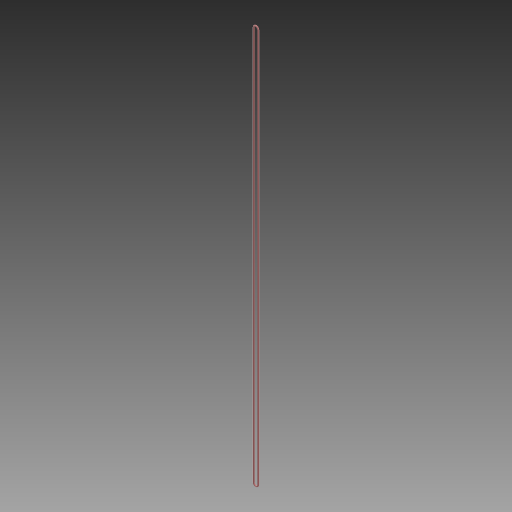
# Autodesk Inventor part: REVLIFT-Test String
Saved by Autodesk Inventor 2023 (Build 270158000, 158)
## iProperties
Created: 2023-01-02
Part Number: REVLIFT-Test String
Material: Nylon 6
Document SubType Name: Modeling
Designer: Max Boord
Mass: 32.7487 g
Surface Area: 292.399 cm^2
Volume: 29.2399 cm^3
Density: 1.12 g/cm^3
Appearance: Smooth - Burnt Red
Author: Max Boord
Autodesk Inventor part; units mm, degrees
ref_plane "YZ Plane" through (0, 0, 0) normal (1, 0, 0) x (0, 1, 0)
ref_plane "XZ Plane" through (0, 0, 0) normal (0, 1, 0) x (-1, 0, 0)
ref_plane "XY Plane" through (0, 0, 0) normal (0, 0, 1) x (1, 0, 0)
sketch "Sketch1" plane through (0, 0, 0) normal (0, 0, 1) x (1, 0, 0)
  line L0 (0, 571.5) -> (0, -571.5) construction
  line L1 (-6.5, 571.5) -> (-6.5, -571.5)
  line L2 (6.5, -571.5) -> (6.5, 571.5)
  arc A0 (6.5, 571.5) -> (-6.5, 571.5) centre (0, 571.5) ccw
  arc A1 (-6.5, -571.5) -> (6.5, -571.5) centre (0, -571.5) ccw
  line L3 (-4.5, 571.5) -> (-4.5, -571.5)
  arc A2 (-4.5, -571.5) -> (4.5, -571.5) centre (0, -571.5) ccw
  line L4 (4.5, -571.5) -> (4.5, 571.5)
  arc A3 (4.5, 571.5) -> (-4.5, 571.5) centre (0, 571.5) ccw
  line L5 (-8.5, 571.5) -> (-8.5, -571.5)
  arc A4 (-8.5, -571.5) -> (8.5, -571.5) centre (0, -571.5) ccw
  line L6 (8.5, -571.5) -> (8.5, 571.5)
  arc A5 (8.5, 571.5) -> (-8.5, 571.5) centre (0, 571.5) ccw
  point P0 (0, 0)
  dimension "d0" = 9
  dimension "d2" = 2
  dimension "d3" = 2
  dimension "d4" = 1143
  constraints: 16 end point, 12 point on circle, 6 centre point, 4 tangent, 3 parallel, 1 midpoint, 1 vertical, 6 other
  measures "d0" diameter of A3
  measures "d2" radial gap between concentric circles of A3 A0
  measures "d3" radial gap between concentric circles of A0 A5
  measures "d4" distance of L0.start L0.end
extrude "Extrusion1" add sketch "Sketch1" along normal mid plane 4 contours A0 L2 A1 L1 | A5 L6 A4 L5
fillet "Fillet1" radius 2 16 edges at (0, -580, 2) (8.5, 0, 2) (0, 580, 2) (-8.5, 0, 2) (0, 576, 2) (4.5, 0, 2) (0, -576, 2) (-4.5, 0, 2) (0, -576, -2) (4.5, 0, -2) (0, 576, -2) (-4.5, 0, -2) (0, 580, -2) (8.5, 0, -2) (0, -580, -2) (-8.5, 0, -2)
body "Solid1"
